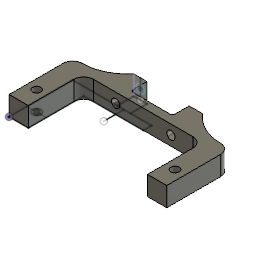
MPU Mount (SEEED ICM) v7 (Autodesk Fusion 360 design; units mm, degrees)
Autodesk Fusion 360 part; units mm, degrees
sketch "Sketch1" plane through (0, 0, 0) normal (0, 1, 0) x (1, 0, 0)
  line L0 (0, 0) -> (0, 23)
  line L1 (0, 23) -> (28.5, 23)
  line L2 (28.5, 23) -> (28.5, 20)
  line L3 (28.5, 20) -> (7, 20)
  line L4 (7, 20) -> (7, 0)
  line L5 (7, 0) -> (0, 0)
  line L6 (7, 6.5) -> (0, 6.5)
  circle A0 centre (3.5, 6.5) radius 1.5
  line L7 (18.5, 23) -> (18.5, 15.7085)
  line L8 (20.9, 23) -> (20.9, 29)
  line L9 (16.1, 23) -> (16.1, 29)
  line L10 (16.1, 29) -> (20.9, 29)
  dimension "d3" = 7
  dimension "d4" = 20
  dimension "d5" = 3
  dimension "d6" = 3
  dimension "d7" = 10
  dimension "d9" = 2.4
  dimension "d10" = 6
  dimension "d19" = 25
  dimension "d22" = 6.5
  constraint coincident L0.start L5.end
  constraint vertical L0
  constraint perpendicular L0 L1
  constraint perpendicular L1 L2
  constraint perpendicular L2 L3
  constraint perpendicular L3 L4
  constraint perpendicular L0 L5
  constraint perpendicular L4 L6
  constraint coincident L0 L6.end
  constraint midpoint L6 A0.centre
  constraint coincident L1 L7.start
  constraint perpendicular L1 L7
  constraint perpendicular L1 L8
  constraint coincident L1 L8.start
  constraint symmetric L7 L8.start L9.start
  constraint symmetric L7 L8.end L9.end
  constraint coincident L4 L6.start
  measures "d3" distance of L4.end L0.start
  measures "d4" distance of L3.end L4.end
  measures "d5" distance of L1.end L2.end
  measures "d6" diameter of A0
  measures "d7" distance of L2 L7
  measures "d9" distance of L7 L8
  measures "d10" distance of L9.start L9.end
  measures "d19" distance of L2 A0.centre
  measures "d22" distance of L5 L6
extrude "Extrude1" add sketch "Sketch1" along normal blind 7 contours L0 L4 L5 L6 A0 | L0 L1 L3 L4 L6 A0 L7 | L1 L8 L9 L10 | L1 L2 L3 L7
chamfer "Chamfer1" distance 6 angle 45 1 edges at (16.1, 3.5, -23)
sketch "Sketch2" plane through (0, 0, -29) normal (0, 0, -1) x (-1, 0, 0)
  line L0 (-20.9, 0) -> (-16.1, 0)
  line L1 (-16.1, 7) -> (-20.9, 7)
  line L2 (-20.9, 7) -> (-20.9, 0)
  line L3 (-18.5, 7) -> (-18.5, 0)
  circle A0 centre (-18.5, 3.5) radius 1.5
  line L4 (-16.1, 0) -> (-16.1, 7)
  dimension "d14" = 3
  constraint midpoint L1 L3.start
  constraint perpendicular L1 L3
  constraint midpoint L3 A0.centre
  measures "d14" diameter of A0
extrude "Extrude2" cut sketch "Sketch2" against normal blind 11 contours L3 A0 | L3 A0
mirror "Mirror1" about plane through (28.5, 0, -23) normal (1, 0, 0) of bodies 1 merged
fillet "Fillet1" radius 3.5 4 edges at (57, 3.5, -23) (0, 3.5, -23) (7, 3.5, -20) (50, 3.5, -20)
fillet "Fillet1" radius 1 2 edges at (36.1, 3.5, -23) (20.9, 3.5, -23)
fillet "Fillet1" radius 16 2 edges at (10.1, 3.5, -23) (46.9, 3.5, -23)
equation "d7 = ( 20 / 2 ) * 1 mm"
equation "d19 = ( 50 / 2 ) * 1 mm"
named bodies: "mpu mnt"
